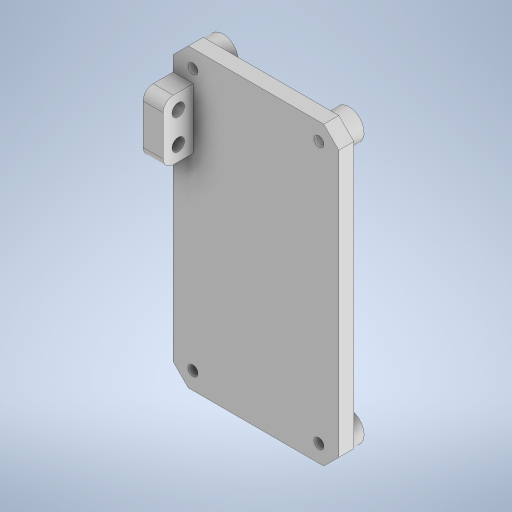
# Autodesk Inventor part: esp커버
Saved by Autodesk Inventor 2023 (Build 270158000, 158)
## iProperties
Created: 2022-08-25
Part Number: esp커버
Material: 일반
Document SubType Name: Modeling
Designer: user
Density: 1 g/cm^3
Appearance: 기본값
Author: user
Autodesk Inventor part; units mm, degrees
ref_plane "YZ Plane" through (0, 0, 0) normal (1, 0, 0) x (0, 1, 0)
ref_plane "XZ Plane" through (0, 0, 0) normal (0, 1, 0) x (-1, 0, 0)
ref_plane "XY Plane" through (0, 0, 0) normal (0, 0, 1) x (1, 0, 0)
sketch "스케치1" plane through (0, 0, 0) normal (0, 0, 1) x (1, 0, 0)
  line L0 (-16.5, -29.5) -> (16.5, -29.5)
  line L1 (16.5, -29.5) -> (16.5, 29.5)
  line L2 (16.5, 29.5) -> (-16.5, 29.5)
  line L3 (-16.5, 29.5) -> (-16.5, -29.5)
  line L4 (-16.5, -29.5) -> (16.5, 29.5) construction
  line L5 (16.5, -29.5) -> (-16.5, 29.5) construction
  line L6 (15.6, -28.8) -> (-15.6, -28.8)
  line L7 (-15.6, -28.8) -> (-15.6, 28.8)
  line L8 (-15.6, 28.8) -> (15.6, 28.8)
  line L9 (15.6, 28.8) -> (15.6, -28.8)
  line L10 (15.6, -28.8) -> (-15.6, 28.8) construction
  line L11 (-15.6, -28.8) -> (15.6, 28.8) construction
  line L12 (0, 0) -> (2, 0)
  line L13 (0, 0) -> (0, 2)
  line L14 (0, 2) -> (0, 5.8071)
  circle A0 centre (-12.55, 26.05) radius 3
  circle A1 centre (12.55, 26.05) radius 3
  circle A2 centre (-12.55, -26.05) radius 3
  circle A3 centre (12.55, -26.05) radius 3
  point P0 (11.351, 28.8)
  point P1 (13.749, 28.8)
  dimension "d0" = 33
  dimension "d1" = 59
  dimension "d8" = 31.2
  dimension "d9" = 57.6
  dimension "d10" = 6
  dimension "d11" = 25.1
  dimension "d12" = 52.1
  dimension "d13" = 2
  dimension "d14" = 2
  dimension "d15" = 3.8071
  constraints: 30 end point, 4 centre point, 4 midpoint, 4 parallel, 3 horizontal, 3 symmetric about line, 2 perpendicular, 1 point on line, 1 vertical, 3 other
  measures "d0" distance of L2.end L1.end
  measures "d1" distance of L1.end L0.end
  measures "d8" distance of L7.end L8.end
  measures "d9" distance of L6.end L7.end
  measures "d10" diameter of A0
  measures "d11" distance of A1.centre A0.centre
  measures "d12" distance of A2.centre A0.centre
  measures "d13" distance of L12.start L13.end
  measures "d14" distance of L12.start L12.end
  measures "d15" distance of L13.end L14.end
extrude "돌출1" add sketch "스케치1" along normal blind 3 contours L3 L2 L1 L0 | L6 A3 A2 L7 L8 A0 A1 L9 | A3 L6 | L6 A3 | A1 L8 | L8 A1 | A2 L6 | L6 A2 | A0 L8 | L8 A0
extrude "돌출2" add sketch "스케치1" against normal blind 3 contours A3 L6 | L6 A3 | A1 L8 | L8 A1 | A2 L6 | L6 A2 | A0 L8 | L8 A0
sketch "스케치3" plane through (-12.55, 26.05, -3) normal (0, 0, -1) x (-1, 0, 0)
  circle A0 centre (0, 0) radius 3 projected
  circle A1 centre (-25.1, 0) radius 3 projected
  circle A2 centre (0, -52.1) radius 3 projected
  circle A3 centre (-25.1, -52.1) radius 3 projected
  point P0 (-12.55, -26.05)
  point P1 (-26.299, 2.75)
  point P2 (-23.901, 2.75)
hole "구멍1" at (-12.55, 26.05, -3) at (12.55, 26.05, -3) at (-12.55, -26.05, -3) at (12.55, -26.05, -3) direction (0, 0, 1) diameter 2 depth 6 countersink diameter 2.5 countersink angle 90
sketch "스케치4" plane through (-16.5, -29.5, 0) normal (-1, 0, 0) x (0, 0, 1)
  line L0 (3, 59) -> (3, 0) projected
  line L1 (9, 41) -> (3, 41)
  line L2 (3, 41) -> (3, 53)
  line L3 (3, 53) -> (9, 53)
  line L4 (9, 53) -> (9, 41)
  line L5 (9, 41) -> (3, 53) construction
  line L6 (3, 41) -> (9, 53) construction
  line L7 (0, 59) -> (3, 59) projected
  circle A0 centre (6, 50) radius 1.25
  line L8 (6, 47) -> (7.5787, 47)
  circle A1 centre (6, 44) radius 1.25
  point P0 (0, 29.5)
  dimension "d27" = 6
  dimension "d28" = 12
  dimension "d29" = 6
  dimension "d32" = 2.5
  dimension "d33" = 6
  constraints: 14 end point, 2 centre point, 2 horizontal, 2 midpoint, 2 parallel, 1 perpendicular, 1 point on line, 1 symmetric about line, 1 other
  measures "d27" distance between parallel lines of L7 L3
  measures "d28" distance of L3.end L1.start
  measures "d29" distance of L2.end L3.end
  measures "d32" diameter of A0
  measures "d33" distance of A1.centre A0.centre
extrude "돌출3" add sketch "스케치4" against normal blind 4
fillet "모깎기1" radius 2 2 edges at (-14.5, 23.5, 9) (-14.5, 11.5, 9)
chamfer "모따기1" distance 3 angle 45 4 edges at (-16.5, 29.5, 1.5) (-16.5, -29.5, 1.5) (16.5, 29.5, 1.5) (16.5, -29.5, 1.5)
